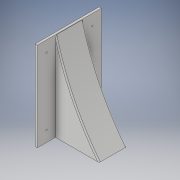
# Autodesk Inventor part: top camera cover
Saved by Autodesk Inventor 2017 (Build 210142000, 142)
## iProperties
Created: 2016-11-05
Part Number: top camera cover
Material: Generic
Document SubType Name: Modeling
Designer: Juan Maldonado
Density: 1 g/cm^3
Appearance: Default
Author: Juan Maldonado
Autodesk Inventor part; units mm, degrees
ref_plane "YZ Plane" through (0, 0, 0) normal (1, 0, 0) x (0, 1, 0)
ref_plane "XZ Plane" through (0, 0, 0) normal (0, 1, 0) x (-1, 0, 0)
ref_plane "XY Plane" through (0, 0, 0) normal (0, 0, 1) x (1, 0, 0)
sketch "Sketch1" plane through (0, 0, 0) normal (0, 0, 1) x (1, 0, 0)
  line L0 (0, 0) -> (127, 0)
  line L1 (0, 0) -> (0, 254)
  arc A0 (0, 254) -> (127, 0) centre (655.239, 422.8695) ccw
  dimension "d0" = 127
  dimension "d1" = 254
  constraints: 4 end point, 2 point on circle, 1 centre point, 1 horizontal, 1 vertical
  measures "d0" distance of L0.start L0.end
  measures "d1" distance of L0.start L1.end
extrude "Extrusion1" add sketch "Sketch1" along normal blind 76.2
fillet "Fillet1" radius 3.175 2 edges at (50.025, 120.2625, 76.2) (50.025, 120.2625, 0)
shell "Shell2" thickness 2.54 removed faces 1 at (0, 161.1309, 50.8)
sketch "Sketch2" plane through (0, 0, 0) normal (0, -1, 0) x (1, 0, 0)
  line L0 (0, 0) -> (127, 0)
  line L1 (127, 0) -> (127, 77.4057)
  line L2 (127, 77.4057) -> (0, 77.4057)
  line L3 (0, 77.4057) -> (0, 0)
  constraints: 8 end point, 2 parallel, 1 horizontal, 1 perpendicular
extrude "Extrusion2" cut sketch "Sketch2" against normal blind 7.9375
sketch "Sketch3" plane through (0, 254, 3.175) normal (-1, 0, 0) x (0, 0, 1)
  line L0 (-53.975, 1.3569) -> (123.825, 1.3569)
  line L1 (123.825, 1.3569) -> (123.825, -245.4504)
  line L2 (123.825, -245.4504) -> (-53.975, -245.4504)
  line L3 (-53.975, -245.4504) -> (-53.975, 1.3569)
  line L4 (-3.175, -12.3037) -> (-3.175, -246.0625) projected
  line L5 (73.025, -246.0625) -> (73.025, -12.3037) projected
  point P0 (-3.175, -254)
  dimension "d13" = 50.8
  dimension "d14" = 50.8
  constraints: 8 end point, 2 parallel, 1 horizontal, 1 perpendicular
  measures "d13" distance between parallel lines of L3 L4
  measures "d14" distance between parallel lines of L5 L1
extrude "Extrusion3" add sketch "Sketch3" along normal blind 6.35
sketch "Sketch5" plane through (0, 254, 3.175) normal (1, 0, 0) x (0, 0, -1)
  circle A0 centre (-98.425, -29.1231) radius 6.35
  circle A1 centre (-98.425, -214.9704) radius 6.35
  line L0 (-123.825, 1.3569) -> (-123.825, -245.4504) projected
  line L1 (53.975, 1.3569) -> (-123.825, 1.3569) projected
  line L2 (-123.825, -245.4504) -> (-73.025, -245.4504) projected
  point P0 (3.175, -254)
  dimension "d15" = 12.7
  dimension "d16" = 12.7
  dimension "d17" = 25.4
  dimension "d35" = 30.48
  dimension "d36" = 30.48
  constraints: 2 centre point, 1 vertical alignment
  measures "d15" diameter of A0
  measures "d16" diameter of A1
  measures "d17" distance from line of L0 A0.centre
  measures "d35" distance from line of A0.centre L1
  measures "d36" distance from line of A1.centre L2
hole "Hole1" at (0, 224.8769, 101.6) at (0, 39.0296, 101.6) direction (-1, 0, 0) diameter 3.6576 end through all
sketch "Sketch6" plane through (0, 254, 3.175) normal (1, 0, 0) x (0, 0, -1)
  circle A0 centre (28.575, -29.1231) radius 6.35
  circle A1 centre (28.575, -214.9704) radius 6.35
  line L0 (53.975, -245.4504) -> (53.975, 1.3569) projected
  line L1 (53.975, 1.3569) -> (-123.825, 1.3569) projected
  line L2 (3.175, -245.4504) -> (53.975, -245.4504) projected
  point P0 (3.175, -254)
  dimension "d25" = 12.7
  dimension "d26" = 12.7
  dimension "d27" = 25.4
  dimension "d37" = 30.48
  dimension "d38" = 30.48
  constraints: 2 centre point, 1 vertical alignment
  measures "d25" diameter of A0
  measures "d26" diameter of A1
  measures "d27" distance from line of A0.centre L0
  measures "d37" distance from line of A0.centre L1
  measures "d38" distance from line of L2 A1.centre
hole "Hole2" at (0, 224.8769, -25.4) at (0, 39.0296, -25.4) direction (-1, 0, 0) diameter 3.6576 end through all
body "Solid1"
